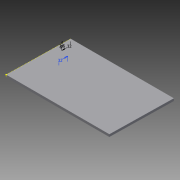
# Autodesk Inventor part: extDisplay
Saved by Autodesk Inventor 2017 (Build 210142000, 142)
## iProperties
Created: 2018-10-12
Part Number: extDisplay
Material: PC/ABS Plastic
Document SubType Name: Modeling
Designer: ari
Density: 0.357273 g/cm^3
Appearance: Smooth - White
Author: ari
Autodesk Inventor part; units mm, degrees
ref_plane "YZ Plane" through (0, 0, 0) normal (1, 0, 0) x (0, 1, 0)
ref_plane "XZ Plane" through (0, 0, 0) normal (0, 1, 0) x (-1, 0, 0)
ref_plane "XY Plane" through (0, 0, 0) normal (0, 0, 1) x (1, 0, 0)
sketch "Sketch1" plane through (0, 0, 0) normal (1, 0, 0) x (0, 1, 0)
  line L0 (0, 0) -> (235.1642, -4.1048)
  line L1 (235.1642, -4.1048) -> (235.0158, -12.6035)
  line L2 (235.0158, -12.6035) -> (-0.1483, -8.4987)
  line L3 (-0.1483, -8.4987) -> (0, 0)
  line L4 (-47.2109, 0) -> (282.2267, 0) construction
  dimension "d0" = 1
  dimension "d1" = 8.5
  dimension "d2" = 235.2
  constraints: 8 end point, 2 parallel, 1 perpendicular
  measures "d0" angle of L0 L4
  measures "d1" distance of L0.end L1.end
  measures "d2" distance of L1.end L2.end
extrude "Extrusion1" add sketch "Sketch1" along normal mid plane 376.2
sketch "Sketch2" plane through (-188.1, 0, 0) normal (-1, 0, 0) x (0, 0, 1)
  line L0 (0, 0) -> (-4.1048, 235.1642) construction
  line L1 (-4.1048, 235.1642) -> (-12.6035, 235.0158) construction
  line L2 (-12.6035, 235.0158) -> (-8.4987, -0.1483) construction
  line L3 (-8.4987, -0.1483) -> (0, 0) construction
  line L4 (-7.7957, 206.2949) -> (-7.7957, 199.8949) construction
  line L5 (-9.0957, 206.2949) -> (-9.0957, 199.8949)
  line L6 (-6.4957, 199.8949) -> (-6.4957, 206.2949)
  arc A0 (-6.4957, 206.2949) -> (-9.0957, 206.2949) centre (-7.7957, 206.2949) ccw
  arc A1 (-9.0957, 199.8949) -> (-6.4957, 199.8949) centre (-7.7957, 199.8949) ccw
  line L7 (-7.7957, 207.5949) -> (-7.7957, 198.5949) construction
  line L8 (-3.545, 203.0949) -> (-12.0463, 203.0949) construction
  point P0 (-7.7957, 203.0949)
  point P1 (-7.7957, 203.0949)
  dimension "d5" = 2.6
  dimension "d6" = 9
  dimension "d7" = 32
  constraints: 12 end point, 6 point on circle, 4 tangent, 3 midpoint, 2 centre point, 2 point on line, 1 horizontal, 1 parallel, 1 vertical
  measures "d5" distance between parallel lines of L5 L6
  measures "d6" distance of L7.start L7.end
  measures "d7" distance from line of L1 point (-7.796, 203.095)
extrude "Extrusion2" cut sketch "Sketch2" against normal blind 10
body "Solid1"
